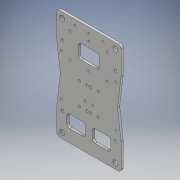
# Autodesk Inventor part: foot_sigmaban_plus
Saved by Autodesk Inventor 2018 (Build 220112000, 112)
## iProperties
Part Number: foot_sigmaban_plus
Material: Générique
Document SubType Name: Modeling
Designer: Gregwar
Density: 1 g/cm^3
Appearance: Par défaut
Vendor: Rhoban
Mass: 36.5439 g
Surface Area: 276.942 cm^2
Volume: 36.5439 cm^3
Author: Gregwar
Autodesk Inventor part; units mm, degrees
ref_plane "YZ Plane" through (0, 0, 0) normal (1, 0, 0) x (0, 1, 0)
ref_plane "XZ Plane" through (0, 0, 0) normal (0, 1, 0) x (-1, 0, 0)
ref_plane "XY Plane" through (0, 0, 0) normal (0, 0, 1) x (1, 0, 0)
sketch "Esquisse1" plane through (0, 0, 0) normal (0, 1, 0) x (-1, 0, 0)
  line L0 (46, 78.8043) -> (-46, 78.8043)
  line L1 (-46, 78.8043) -> (-46, -78.8043)
  line L2 (-46, -78.8043) -> (46, -78.8043)
  line L3 (46, -78.8043) -> (46, 78.8043)
  line L4 (0, 78.8043) -> (0, -78.8043) construction
  line L5 (46, 0) -> (-46, 0) construction
  line L6 (38, 78.8043) -> (38, -78.8043) construction
  circle A0 centre (38, 70.8043) radius 3.65
  circle A1 centre (38, 43.8043) radius 2
  line L7 (38, -78.8043) -> (38, 78.8043) construction
  circle A2 centre (38, -70.8043) radius 3.65
  circle A3 centre (38, -43.8043) radius 2
  line L8 (-38, 78.8043) -> (-38, -78.8043) construction
  circle A4 centre (-38, 70.8043) radius 3.65
  circle A5 centre (-38, 43.8043) radius 2
  line L9 (-38, -78.8043) -> (-38, 78.8043) construction
  circle A6 centre (-38, -70.8043) radius 3.65
  circle A7 centre (-38, -43.8043) radius 2
  point P0 (0, 0)
  point P1 (0, 0)
  dimension "d0" = 7.3
  dimension "d1" = 4
  dimension "d2" = 8
  dimension "d3" = 8
  dimension "d6" = 27
  dimension "d55" = 92
  dimension "d56" = 157.6087
  dimension "d61" = 76
  dimension "d62" = 141.6087
  constraints: 20 end point, 12 symmetric about line, 10 point on line, 8 centre point, 5 midpoint, 2 parallel, 2 perpendicular, 1 coincident, 1 horizontal, 6 other
  measures "d0" diameter of A0
  measures "d1" diameter of A1
  measures "d2" distance from line of L0 A0.centre
  measures "d3" distance from line of L3 A0.centre
  measures "d6" distance of A1.centre A0.centre
  measures "d55" distance of L1.end L2.end
  measures "d56" distance between parallel lines of L0 L2
  measures "d61" distance of A4.centre A0.centre
  measures "d62" distance of A6.centre A4.centre
extrude "Extrusion1" add sketch "Esquisse1" along normal blind 3
sketch "Esquisse2" plane through (0, 3, 0) normal (0, 1, 0) x (1, 0, 0)
  line L0 (-2.5, -5.5) -> (13.5, -5.5) construction
  line L1 (13.5, -5.5) -> (13.5, 26.5) construction
  line L2 (13.5, 26.5) -> (-2.5, 26.5) construction
  line L3 (-2.5, 26.5) -> (-2.5, -5.5) construction
  line L4 (-46, -78.8043) -> (46, -78.8043) construction
  line L5 (0, -78.8043) -> (0, 78.8043) construction
  line L6 (46, 78.8043) -> (-46, 78.8043) construction
  line L7 (-46, 78.8043) -> (-46, -78.8043) construction
  line L8 (-46, 0) -> (46, 0) construction
  line L9 (46, -78.8043) -> (46, 78.8043) construction
  line L10 (-2.5, 10.5) -> (13.5, 10.5) construction
  line L11 (5.5, -5.5) -> (5.5, 26.5) construction
  circle A0 centre (-2.5, -5.5) radius 1.5
  circle A1 centre (13.5, -5.5) radius 1.5
  circle A2 centre (13.5, 26.5) radius 1.5
  circle A3 centre (-2.5, 26.5) radius 1.5
  line L12 (-2.5, 15.5) -> (13.5, 15.5) construction
  circle A4 centre (5.5, 15.5) radius 1.5
  line L13 (2.5, -5.5) -> (-13.5, -5.5) construction
  line L14 (-13.5, -5.5) -> (-13.5, 26.5) construction
  line L15 (-13.5, 26.5) -> (2.5, 26.5) construction
  line L16 (2.5, 26.5) -> (2.5, -5.5) construction
  line L17 (2.5, 10.5) -> (-13.5, 10.5) construction
  line L18 (-5.5, -5.5) -> (-5.5, 26.5) construction
  circle A5 centre (2.5, -5.5) radius 1.5
  circle A6 centre (-13.5, -5.5) radius 1.5
  circle A7 centre (-13.5, 26.5) radius 1.5
  circle A8 centre (2.5, 26.5) radius 1.5
  line L19 (2.5, 15.5) -> (-13.5, 15.5) construction
  circle A9 centre (-5.5, 15.5) radius 1.5
  circle A10 centre (-38, 70.8043) radius 3.65 projected
  line L20 (-46, -20.5) -> (46, -20.5) construction
  circle A11 centre (38, 43.8043) radius 2 construction
  circle A12 centre (38, 70.8043) radius 3.65 projected
  point P0 (0, 0)
  dimension "d9" = 32
  dimension "d10" = 16
  dimension "d14" = 3
  dimension "d17" = 5
  dimension "d28" = 10.5
  dimension "d29" = 15
  dimension "d54" = 32.5
  dimension "d63" = 55.3043
  constraints: 34 end point, 15 symmetric about line, 10 centre point, 9 midpoint, 8 coincident, 6 point on line, 4 equal radius, 2 horizontal, 2 parallel, 2 perpendicular, 5 other
  measures "d9" distance of L2.end L0.start
  measures "d10" distance of L1.end L2.end
  measures "d14" diameter of A0
  measures "d17" distance between parallel lines of L17 L19
  measures "d28" distance between parallel lines of L8 L17
  measures "d29" distance from line of L20 A6.centre
  measures "d54" distance from line of L11 A11.centre
  measures "d63" vertical distance of A4.centre A12.centre
extrude "Extrusion2" cut sketch "Esquisse2" against normal through all contours A0 | A1 | A2 | A3 | A4 | A5 | A6 | A7 | A8 | A9
sketch "Esquisse4" plane through (0, 3, 0) normal (0, 1, 0) x (1, 0, 0)
  circle A0 centre (-5.5, 15.5) radius 1.5 construction
  circle A1 centre (2.5, 26.5) radius 1.5 construction
  circle A2 centre (5.5, 15.5) radius 1.5 construction
  circle A3 centre (13.5, 26.5) radius 1.5 construction
  circle A4 centre (-2.5, -5.5) radius 1.5 construction
  circle A5 centre (13.5, -5.5) radius 1.5 construction
  circle A6 centre (-2.5, 26.5) radius 1.5 construction
  circle A7 centre (2.5, -5.5) radius 1.5 construction
  circle A8 centre (-13.5, 26.5) radius 1.5 construction
  circle A9 centre (-13.5, -5.5) radius 1.5 construction
  circle A10 centre (38, 70.8043) radius 3.65 construction
  circle A11 centre (38, -70.8043) radius 3.65 construction
  circle A12 centre (-38, 70.8043) radius 3.65 construction
  circle A13 centre (-38, -70.8043) radius 3.65 construction
  circle A14 centre (38, 43.8043) radius 2 construction
  circle A15 centre (38, -43.8043) radius 2 construction
  circle A16 centre (-38, 43.8043) radius 2 construction
  circle A17 centre (-38, -43.8043) radius 2 construction
  line L0 (-46, -78.8043) -> (46, -78.8043) construction
  line L1 (46, -78.8043) -> (46, 78.8043) construction
  line L2 (46, 78.8043) -> (-46, 78.8043) construction
  line L3 (-46, 78.8043) -> (-46, -78.8043) construction
  line L4 (0, -78.8043) -> (0, 0) construction
  line L5 (30, -64.3043) -> (-30, -64.3043) construction
  line L6 (-30, -64.3043) -> (-30, -21.3043) construction
  line L7 (-30, -21.3043) -> (30, -21.3043) construction
  line L8 (30, -21.3043) -> (30, -64.3043) construction
  line L9 (0, -64.3043) -> (0, -21.3043) construction
  line L10 (30, -61.0043) -> (-30, -61.0043) construction
  line L11 (30, -42.8043) -> (-30, -42.8043) construction
  line L12 (30, -24.6043) -> (-30, -24.6043) construction
  circle A18 centre (26.5, -61.0043) radius 1.5
  circle A19 centre (0, -61.0043) radius 1.5
  circle A20 centre (-26.5, -61.0043) radius 1.5
  circle A21 centre (26.5, -24.6043) radius 1.5
  circle A22 centre (0, -24.6043) radius 1.5
  circle A23 centre (-26.5, -24.6043) radius 1.5
  line L13 (46, -18.5) -> (-46, -18.5) construction
  dimension "d18" = 60
  dimension "d19" = 43
  dimension "d20" = 14.5
  dimension "d21" = 3.3
  dimension "d22" = 3
  dimension "d23" = 53
  dimension "d57" = 13
  constraints: 20 end point, 6 centre point, 6 midpoint, 6 symmetric about line, 5 point on line, 2 horizontal, 2 parallel, 2 perpendicular, 1 collinear, 1 equal radius, 1 vertical, 4 other
  measures "d18" distance of L5.start L5.end
  measures "d19" distance of L5.end L6.end
  measures "d20" distance between parallel lines of L0 L5
  measures "d21" distance between parallel lines of L5 L10
  measures "d22" diameter of A20
  measures "d23" distance of A18.centre A20.centre
  measures "d57" distance from line of L13 A5.centre
extrude "Extrusion3" cut sketch "Esquisse4" against normal through all
fillet "Congé1" radius 4 4 edges at (46, 1.5, -78.8043) (-46, 1.5, -78.8043) (-46, 1.5, 78.8043) (46, 1.5, 78.8043)
sketch "Esquisse6" plane through (0, 3, 0) normal (0, 1, 0) x (1, 0, 0)
  arc A0 (42, -78.8043) -> (46, -74.8043) centre (42, -74.8043) ccw construction
  line L0 (46, -74.8043) -> (46, 74.8043) construction
  arc A1 (46, 74.8043) -> (42, 78.8043) centre (42, 74.8043) ccw construction
  line L1 (42, 78.8043) -> (-42, 78.8043) construction
  arc A2 (-42, 78.8043) -> (-46, 74.8043) centre (-42, 74.8043) ccw construction
  line L2 (-46, 74.8043) -> (-46, -74.8043) construction
  arc A3 (-46, -74.8043) -> (-42, -78.8043) centre (-42, -74.8043) ccw construction
  line L3 (-42, -78.8043) -> (42, -78.8043) construction
  circle A4 centre (26.5, -24.6043) radius 1.5 construction
  circle A5 centre (-26.5, -61.0043) radius 1.5 construction
  circle A6 centre (26.5, -61.0043) radius 1.5 construction
  circle A7 centre (0, -61.0043) radius 1.5 construction
  circle A8 centre (-26.5, -24.6043) radius 1.5 construction
  circle A9 centre (0, -24.6043) radius 1.5 construction
  circle A10 centre (-5.5, 15.5) radius 1.5 construction
  circle A11 centre (2.5, 26.5) radius 1.5 construction
  circle A12 centre (5.5, 15.5) radius 1.5 construction
  circle A13 centre (13.5, 26.5) radius 1.5 construction
  circle A14 centre (-2.5, -5.5) radius 1.5 construction
  circle A15 centre (13.5, -5.5) radius 1.5 construction
  circle A16 centre (-2.5, 26.5) radius 1.5 construction
  circle A17 centre (2.5, -5.5) radius 1.5 construction
  circle A18 centre (-13.5, 26.5) radius 1.5 construction
  circle A19 centre (-13.5, -5.5) radius 1.5 construction
  circle A20 centre (38, 70.8043) radius 3.65 construction
  circle A21 centre (38, -70.8043) radius 3.65 construction
  circle A22 centre (-38, 70.8043) radius 3.65 construction
  circle A23 centre (-38, -70.8043) radius 3.65 construction
  circle A24 centre (38, 43.8043) radius 2 construction
  circle A25 centre (38, -43.8043) radius 2 construction
  circle A26 centre (-38, 43.8043) radius 2 construction
  circle A27 centre (-38, -43.8043) radius 2 construction
  line L4 (-46, 0) -> (-41, 0) construction
  line L5 (-46, -40) -> (-41, 0)
  line L6 (-41, 0) -> (-46, 40)
  line L7 (-46, 40) -> (-46, -40)
  line L8 (-46, 74.8043) -> (-46, -74.8043) projected
  line L9 (0, -78.8043) -> (0, 78.8043) construction
  line L10 (42, 78.8043) -> (-42, 78.8043) construction
  line L11 (46, 0) -> (41, 0) construction
  line L12 (46, -40) -> (41, 0)
  line L13 (41, 0) -> (46, 40)
  line L14 (46, 40) -> (46, -40)
  line L15 (-15, -53.0043) -> (15, -53.0043)
  line L16 (15, -53.0043) -> (15, -32.6043)
  line L17 (15, -32.6043) -> (-15, -32.6043)
  line L18 (-15, -32.6043) -> (-15, -53.0043)
  line L19 (-31.5, 42.8043) -> (31.5, 42.8043)
  line L20 (31.5, 42.8043) -> (31.5, 60.8043)
  line L21 (31.5, 60.8043) -> (-31.5, 60.8043)
  line L22 (-31.5, 60.8043) -> (-31.5, 42.8043)
  line L23 (38, -70.8043) -> (-38, -70.8043) construction
  circle A28 centre (0, -70.8043) radius 1.5
  circle A29 centre (20, -70.8043) radius 1.5
  circle A30 centre (-20, -70.8043) radius 1.5
  point P0 (0, 0)
  point P1 (0, -53)
  point P2 (0, -32.6043)
  point P3 (0, 42.8043)
  dimension "d30" = 5
  dimension "d31" = 80
  dimension "d35" = 8
  dimension "d36" = 8
  dimension "d37" = 30
  dimension "d38" = 18
  dimension "d39" = 18
  dimension "d58" = 3
  dimension "d59" = 20
  constraints: 36 end point, 6 midpoint, 6 point on line, 5 symmetric about line, 4 horizontal, 4 parallel, 3 centre point, 2 perpendicular, 1 collinear, 1 equal length, 1 equal radius, 1 other
  measures "d30" distance of L4.start L4.end
  measures "d31" distance of L5.start L6.end
  measures "d35" distance from line of A5.centre L15
  measures "d36" distance from line of A9.centre L17
  measures "d37" distance of L16.end L17.end
  measures "d38" distance between parallel lines of L21 L1
  measures "d39" distance of L21.end L19.start
  measures "d58" diameter of A29
  measures "d59" distance of A29.centre A28.centre
extrude "Extrusion4" cut sketch "Esquisse6" against normal through all
sketch "Esquisse7" plane through (0, 3, 0) normal (0, 1, 0) x (1, 0, 0)
  circle A0 centre (-38, -43.8043) radius 2 construction
  circle A1 centre (-38, 43.8043) radius 2 construction
  circle A2 centre (38, -43.8043) radius 2 construction
  circle A3 centre (38, 43.8043) radius 2 construction
  circle A4 centre (-38, -70.8043) radius 3.65 construction
  circle A5 centre (-38, 70.8043) radius 3.65 construction
  circle A6 centre (38, -70.8043) radius 3.65 construction
  circle A7 centre (38, 70.8043) radius 3.65 construction
  circle A8 centre (-13.5, -5.5) radius 1.5 construction
  circle A9 centre (-13.5, 26.5) radius 1.5 construction
  circle A10 centre (2.5, -5.5) radius 1.5 construction
  circle A11 centre (-2.5, 26.5) radius 1.5 construction
  circle A12 centre (13.5, -5.5) radius 1.5 construction
  circle A13 centre (-2.5, -5.5) radius 1.5 construction
  circle A14 centre (13.5, 26.5) radius 1.5 construction
  circle A15 centre (5.5, 15.5) radius 1.5 construction
  circle A16 centre (2.5, 26.5) radius 1.5 construction
  circle A17 centre (-5.5, 15.5) radius 1.5 construction
  circle A18 centre (0, -24.6043) radius 1.5 construction
  circle A19 centre (-26.5, -24.6043) radius 1.5 construction
  circle A20 centre (0, -61.0043) radius 1.5 construction
  circle A21 centre (26.5, -61.0043) radius 1.5 construction
  circle A22 centre (-26.5, -61.0043) radius 1.5 construction
  circle A23 centre (26.5, -24.6043) radius 1.5 construction
  line L0 (31.5, 60.8043) -> (31.5, 42.8043) construction
  line L1 (31.5, 42.8043) -> (-31.5, 42.8043) construction
  line L2 (-31.5, 42.8043) -> (-31.5, 60.8043) construction
  line L3 (-31.5, 60.8043) -> (31.5, 60.8043) construction
  line L4 (15, -32.6043) -> (15, -53.0043) construction
  line L5 (15, -53.0043) -> (-15, -53.0043) construction
  line L6 (-15, -53.0043) -> (-15, -32.6043) construction
  line L7 (-15, -32.6043) -> (15, -32.6043) construction
  line L8 (46, -40) -> (41, 0) construction
  line L9 (41, 0) -> (46, 40) construction
  line L10 (46, 40) -> (46, 74.8043) construction
  arc A24 (46, 74.8043) -> (42, 78.8043) centre (42, 74.8043) ccw construction
  line L11 (42, 78.8043) -> (-42, 78.8043) construction
  arc A25 (-42, 78.8043) -> (-46, 74.8043) centre (-42, 74.8043) ccw construction
  line L12 (-46, 74.8043) -> (-46, 40) construction
  line L13 (-46, 40) -> (-41, 0) construction
  line L14 (-41, 0) -> (-46, -40) construction
  line L15 (-46, -40) -> (-46, -74.8043) construction
  arc A26 (-46, -74.8043) -> (-42, -78.8043) centre (-42, -74.8043) ccw construction
  line L16 (-42, -78.8043) -> (42, -78.8043) construction
  arc A27 (42, -78.8043) -> (46, -74.8043) centre (42, -74.8043) ccw construction
  line L17 (46, -74.8043) -> (46, -40) construction
  line L18 (-5, 42.8043) -> (5, 42.8043)
  line L19 (5, 42.8043) -> (5, 60.8043)
  line L20 (5, 60.8043) -> (-5, 60.8043)
  line L21 (-5, 60.8043) -> (-5, 42.8043)
  point P0 (0, 0)
  point P1 (0, 60.8043)
  point P2 (0, 42.8043)
  dimension "d43" = 10
  constraints: 8 end point, 4 midpoint, 2 parallel, 1 horizontal, 1 perpendicular
  measures "d43" distance between parallel lines of L19 L21
extrude "Extrusion5" add sketch "Esquisse7" against normal blind 3
fillet "Congé2" radius 4 12 edges at (-31.5, 1.5, -60.8043) (5, 1.5, -60.8043) (-15, 1.5, 32.6043) (-15, 1.5, 53.0043) (-31.5, 1.5, -42.8043) (5, 1.5, -42.8043) (15, 1.5, 53.0043) (-5, 1.5, -42.8043) (31.5, 1.5, -42.8043) (-5, 1.5, -60.8043) (31.5, 1.5, -60.8043) (15, 1.5, 32.6043)
fillet "Congé3" radius 10 6 edges at (-46, 1.5, 40) (-41, 1.5, 0) (-46, 1.5, -40) (46, 1.5, -40) (41, 1.5, 0) (46, 1.5, 40)
sketch "Esquisse8" plane through (0, 3, 0) normal (0, 1, 0) x (1, 0, 0)
  line L0 (9, 60.8043) -> (27.5, 60.8043) construction
  arc A0 (31.5, 56.8043) -> (27.5, 60.8043) centre (27.5, 56.8043) ccw construction
  line L1 (31.5, 56.8043) -> (31.5, 46.8043) construction
  line L2 (27.5, 42.8043) -> (9, 42.8043) construction
  circle A1 centre (-38, -43.8043) radius 2 construction
  circle A2 centre (-38, 43.8043) radius 2 construction
  circle A3 centre (38, -43.8043) radius 2 construction
  circle A4 centre (38, 43.8043) radius 2 construction
  circle A5 centre (-38, -70.8043) radius 3.65 construction
  circle A6 centre (-38, 70.8043) radius 3.65 construction
  circle A7 centre (38, -70.8043) radius 3.65 construction
  circle A8 centre (38, 70.8043) radius 3.65 construction
  circle A9 centre (-13.5, -5.5) radius 1.5 construction
  circle A10 centre (-13.5, 26.5) radius 1.5 construction
  circle A11 centre (2.5, -5.5) radius 1.5 construction
  circle A12 centre (-2.5, 26.5) radius 1.5 construction
  circle A13 centre (13.5, -5.5) radius 1.5 construction
  circle A14 centre (-2.5, -5.5) radius 1.5 construction
  circle A15 centre (13.5, 26.5) radius 1.5 construction
  circle A16 centre (5.5, 15.5) radius 1.5 construction
  circle A17 centre (2.5, 26.5) radius 1.5 construction
  circle A18 centre (-5.5, 15.5) radius 1.5 construction
  circle A19 centre (0, -24.6043) radius 1.5 construction
  circle A20 centre (-26.5, -24.6043) radius 1.5 construction
  circle A21 centre (26.5, -61.0043) radius 1.5 construction
  circle A22 centre (-26.5, -61.0043) radius 1.5 construction
  circle A23 centre (26.5, -24.6043) radius 1.5 construction
  line L3 (-31.5, 46.8043) -> (-31.5, 56.8043) construction
  arc A24 (-27.5, 60.8043) -> (-31.5, 56.8043) centre (-27.5, 56.8043) ccw construction
  line L4 (15, -36.6043) -> (15, -49.0043) construction
  arc A25 (11, -53.0043) -> (15, -49.0043) centre (11, -49.0043) ccw construction
  line L5 (11, -53.0043) -> (-11, -53.0043) construction
  arc A26 (-15, -49.0043) -> (-11, -53.0043) centre (-11, -49.0043) ccw construction
  line L6 (-15, -49.0043) -> (-15, -36.6043) construction
  arc A27 (-11, -32.6043) -> (-15, -36.6043) centre (-11, -36.6043) ccw construction
  line L7 (-11, -32.6043) -> (11, -32.6043) construction
  arc A28 (15, -36.6043) -> (11, -32.6043) centre (11, -36.6043) ccw construction
  arc A29 (46, -40.6226) -> (45.9228, -39.3822) centre (36, -40.6226) ccw construction
  line L8 (45.9228, -39.3822) -> (41.155, -1.2403) construction
  arc A30 (41.155, 1.2403) -> (41.155, -1.2403) centre (51.0778, 0) ccw construction
  line L9 (41.155, 1.2403) -> (45.9228, 39.3822) construction
  arc A31 (45.9228, 39.3822) -> (46, 40.6226) centre (36, 40.6226) ccw construction
  line L10 (46, 40.6226) -> (46, 74.8043) construction
  arc A32 (46, 74.8043) -> (42, 78.8043) centre (42, 74.8043) ccw construction
  line L11 (42, 78.8043) -> (-42, 78.8043) construction
  arc A33 (-42, 78.8043) -> (-46, 74.8043) centre (-42, 74.8043) ccw construction
  line L12 (-46, 74.8043) -> (-46, 40.6226) construction
  arc A34 (-46, 40.6226) -> (-45.9228, 39.3822) centre (-36, 40.6226) ccw construction
  line L13 (-45.9228, 39.3822) -> (-41.155, 1.2403) construction
  arc A35 (-41.155, -1.2403) -> (-41.155, 1.2403) centre (-51.0778, 0) ccw construction
  line L14 (-41.155, -1.2403) -> (-45.9228, -39.3822) construction
  arc A36 (-45.9228, -39.3822) -> (-46, -40.6226) centre (-36, -40.6226) ccw construction
  line L15 (-46, -40.6226) -> (-46, -74.8043) construction
  arc A37 (-46, -74.8043) -> (-42, -78.8043) centre (-42, -74.8043) ccw construction
  line L16 (-42, -78.8043) -> (42, -78.8043) construction
  arc A38 (42, -78.8043) -> (46, -74.8043) centre (42, -74.8043) ccw construction
  line L17 (46, -74.8043) -> (46, -40.6226) construction
  line L18 (-39, -78.8043) -> (-39, 78.8043) construction
  line L19 (42, 78.8043) -> (-42, 78.8043) construction
  line L20 (42, 78.8043) -> (-42, 78.8043) construction
  line L21 (0, -78.8043) -> (0, 78.8043) construction
  line L22 (39, -78.8043) -> (39, 78.8043) construction
  line L23 (0, 0) -> (-39, 0) construction
  circle A39 centre (-39, -30) radius 1.5
  circle A40 centre (-39, 30) radius 1.5
  circle A41 centre (39, -30) radius 1.5
  circle A42 centre (39, 30) radius 1.5
  arc A43 (5, 46.8043) -> (9, 42.8043) centre (9, 46.8043) ccw projected
  line L24 (5, 46.8043) -> (5, 56.8043) projected
  arc A44 (9, 60.8043) -> (5, 56.8043) centre (9, 56.8043) ccw projected
  line L25 (-5, 56.8043) -> (-5, 46.8043) projected
  arc A45 (-9, 42.8043) -> (-5, 46.8043) centre (-9, 46.8043) ccw projected
  line L26 (-27.5, 60.8043) -> (-9, 60.8043) projected
  arc A46 (-5, 56.8043) -> (-9, 60.8043) centre (-9, 56.8043) ccw projected
  arc A47 (27.5, 42.8043) -> (31.5, 46.8043) centre (27.5, 46.8043) ccw projected
  line L27 (-9, 42.8043) -> (-27.5, 42.8043) projected
  arc A48 (-31.5, 46.8043) -> (-27.5, 42.8043) centre (-27.5, 46.8043) ccw projected
  point P0 (39, 0)
  dimension "d49" = 7
  dimension "d50" = 30
  dimension "d51" = 3
  constraints: 8 end point, 6 symmetric about line, 4 centre point, 3 midpoint, 3 point on line, 1 perpendicular, 3 other
  measures "d49" distance between parallel lines of L18 L15
  measures "d50" distance from line of L23 A39.centre
  measures "d51" diameter of A39
extrude "Extrusion6" cut sketch "Esquisse8" against normal through all
equation "\"d3\" = d2"
equation "\"d36\" = d35"
